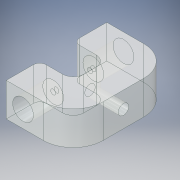
# Autodesk Inventor part: lickPort1
Saved by Autodesk Inventor 2019 (Build 230136000, 136)
## iProperties
Created: 2019-01-07
Part Number: lickPort1
Material: Generic
Document SubType Name: Modeling
Designer: Brian
Density: 1 g/cm^3
Appearance: Clear
Author: Brian
Autodesk Inventor part; units mm, degrees
ref_plane "YZ Plane" through (0, 0, 0) normal (1, 0, 0) x (0, 1, 0)
ref_plane "XZ Plane" through (0, 0, 0) normal (0, 1, 0) x (-1, 0, 0)
ref_plane "XY Plane" through (0, 0, 0) normal (0, 0, 1) x (1, 0, 0)
sketch "Sketch1" plane through (0, 0, 0) normal (0, 1, 0) x (-1, 0, 0)
  line L0 (0, 0) -> (20, 0)
  line L1 (20, -30) -> (0, -30)
  line L2 (0, -30) -> (0, 0)
  line L3 (20, 0) -> (20, -10)
  line L4 (20, -10) -> (10, -10)
  line L5 (10, -10) -> (10, -20)
  line L6 (10, -20) -> (20, -20)
  line L7 (20, -20) -> (20, -30)
  dimension "d0" = 20
  dimension "d1" = 30
  dimension "d2" = 10
  dimension "d3" = 10
  dimension "d4" = 10
  dimension "d5" = 10
  dimension "d8" = 20
  constraints: 16 end point, 3 perpendicular, 1 horizontal, 1 parallel, 1 point on line, 1 vertical
  measures "d0" distance of L1.start L1.end
  measures "d1" distance of L0.end L1.start
  measures "d2" distance of L0.end L3.end
  measures "d3" distance of L3.end L4.end
  measures "d4" distance of L4.end L5.end
  measures "d5" distance of L5.end L6.end
  measures "d8" distance of L0.start L0.end
extrude "Extrusion1" add sketch "Sketch1" along normal blind 10
sketch "Sketch2" plane through (-20, 0, 0) normal (0, 0, 1) x (1, 0, 0)
  line L0 (0, 0) -> (0, 10) projected
  line L1 (0, 10) -> (20, 10) projected
  point P0 (20, 0)
  point P1 (5, 5)
  dimension "d16" = 5
  dimension "d17" = 5
  measures "d16" distance from line of L0 point (5, 5)
  measures "d17" distance from line of L1 point (5, 5)
hole "Hole1" at (-15, 5, 0) direction (0, 0, -1) diameter 1.5 depth 11 counterbore diameter 6.2 counterbore depth 9
sketch "Sketch3" plane through (0, 0, -30) normal (0, 0, -1) x (-1, 0, 0)
  line L0 (20, 0) -> (20, 10) projected
  line L1 (0, 10) -> (20, 10) projected
  point P0 (0, 0)
  point P1 (15, 5)
  dimension "d25" = 5
  dimension "d26" = 5
  measures "d25" distance from line of L0 point (15, 5)
  measures "d26" distance from line of L1 point (15, 5)
hole "Hole2" at (-15, 5, -30) direction (0, 0, 1) diameter 1.5 depth 11 counterbore diameter 6.2 counterbore depth 9
sketch "Sketch4" plane through (0, 0, 0) normal (1, 0, 0) x (0, 0, -1)
  line L0 (0, 10) -> (30, 10) projected
  line L1 (30, 0) -> (30, 10) projected
  point P0 (0, 0)
  point P1 (15, 5)
  dimension "d34" = 5
  dimension "d35" = 15
  measures "d34" distance from line of L0 point (15, 5)
  measures "d35" distance from line of L1 point (15, 5)
hole "Hole3" at (0, 5, -15) direction (-1, 0, 0) diameter 3.1 depth 20
fillet "Fillet1" radius 3.175 1 edges at (-10, 5, -20)
fillet "Fillet2" radius 3.175 1 edges at (-10, 5, -10)
fillet "Fillet3" radius 1.905 1 edges at (-20, 5, -20)
fillet "Fillet4" radius 1.905 1 edges at (-20, 5, -10)
fillet "Fillet5" radius 8.89 1 edges at (0, 5, -30)
fillet "Fillet6" radius 8.89 1 edges at (0, 5, 0)
body "Solid1"
